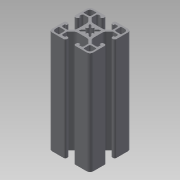
# Autodesk Inventor part: 40-4040-UL
Saved by Autodesk Inventor 2013 (Build 170138000, 138)
## iProperties
Created: 2014-04-23
Part Number: 40-4040-UL
Material: Generic
Document SubType Name: Modeling
Designer: Ross Bowman
Density: 1 g/cm^3
Engineer: Ross Bowman
Catalog Web Link: 8020.net
Vendor: 80/20 Inc.
Company: 80/20 Inc.
Author: Ross Bowman
Keywords: 80/20 , 8020 , T-Slot , Extrusion
Material: 6105-T5 Aluminum
Autodesk Inventor part; units mm, degrees
ref_plane "YZ Plane" through (0, 0, 0) normal (1, 0, 0) x (0, 1, 0)
ref_plane "XZ Plane" through (0, 0, 0) normal (0, 1, 0) x (-1, 0, 0)
ref_plane "XY Plane" through (0, 0, 0) normal (0, 0, 1) x (1, 0, 0)
sketch "Sketch1" plane through (0, 0, 0) normal (0, 0, 1) x (1, 0, 0)
  arc A0 (-5.4393, -4.8481) -> (-4.8481, -5.4393) centre (-4.9497, -4.9497) ccw
  line L0 (-5.1263, -3.712) -> (-5.4393, -4.8481)
  line L1 (-3.0049, -1.5907) -> (-5.1263, -3.712)
  arc A1 (-3.3421, -0.625) -> (-3.0049, -1.5907) centre (0, 0) ccw
  line L2 (-4.0876, -0.4923) -> (-3.3421, -0.625)
  arc A2 (-4.0876, 0.4923) -> (-4.0876, -0.4923) centre (-4, 0) ccw
  line L3 (-3.3421, 0.625) -> (-4.0876, 0.4923)
  arc A3 (-3.0049, 1.5907) -> (-3.3421, 0.625) centre (0, 0) ccw
  line L4 (-5.1263, 3.712) -> (-3.0049, 1.5907)
  line L5 (-5.4393, 4.8481) -> (-5.1263, 3.712)
  arc A4 (-4.8481, 5.4393) -> (-5.4393, 4.8481) centre (-4.9497, 4.9497) ccw
  line L6 (-3.712, 5.1263) -> (-4.8481, 5.4393)
  line L7 (-1.5907, 3.0049) -> (-3.712, 5.1263)
  arc A5 (-0.625, 3.3421) -> (-1.5907, 3.0049) centre (0, 0) ccw
  line L8 (-0.4923, 4.0876) -> (-0.625, 3.3421)
  arc A6 (0.4923, 4.0876) -> (-0.4923, 4.0876) centre (0, 4) ccw
  line L9 (0.625, 3.3421) -> (0.4923, 4.0876)
  arc A7 (1.5907, 3.0049) -> (0.625, 3.3421) centre (0, 0) ccw
  line L10 (3.712, 5.1263) -> (1.5907, 3.0049)
  line L11 (4.8481, 5.4393) -> (3.712, 5.1263)
  arc A8 (5.4393, 4.8481) -> (4.8481, 5.4393) centre (4.9497, 4.9497) ccw
  line L12 (5.1263, 3.712) -> (5.4393, 4.8481)
  line L13 (3.0049, 1.5907) -> (5.1263, 3.712)
  arc A9 (3.3421, 0.625) -> (3.0049, 1.5907) centre (0, 0) ccw
  line L14 (4.0876, 0.4923) -> (3.3421, 0.625)
  arc A10 (4.0876, -0.4923) -> (4.0876, 0.4923) centre (4, 0) ccw
  line L15 (3.3421, -0.625) -> (4.0876, -0.4923)
  arc A11 (3.0049, -1.5907) -> (3.3421, -0.625) centre (0, 0) ccw
  line L16 (5.1263, -3.712) -> (3.0049, -1.5907)
  line L17 (5.4393, -4.8481) -> (5.1263, -3.712)
  arc A12 (4.8481, -5.4393) -> (5.4393, -4.8481) centre (4.9497, -4.9497) ccw
  line L18 (3.712, -5.1263) -> (4.8481, -5.4393)
  line L19 (1.5907, -3.0049) -> (3.712, -5.1263)
  arc A13 (0.625, -3.3421) -> (1.5907, -3.0049) centre (0, 0) ccw
  line L20 (0.4923, -4.0876) -> (0.625, -3.3421)
  arc A14 (-0.4923, -4.0876) -> (0.4923, -4.0876) centre (0, -4) ccw
  line L21 (-0.625, -3.3421) -> (-0.4923, -4.0876)
  arc A15 (-1.5907, -3.0049) -> (-0.625, -3.3421) centre (0, 0) ccw
  line L22 (-3.712, -5.1263) -> (-1.5907, -3.0049)
  line L23 (-4.8481, -5.4393) -> (-3.712, -5.1263)
  arc A16 (-15.545, 18.345) -> (-18.345, 15.545) centre (-15.545, 15.545) ccw
  line L24 (-12.4898, 18.345) -> (-15.545, 18.345)
  arc A17 (-11.8598, 17.715) -> (-12.4898, 18.345) centre (-12.4898, 17.715) ccw
  line L25 (-11.8598, 13.1298) -> (-11.8598, 17.715)
  arc A18 (-13.1298, 11.8598) -> (-11.8598, 13.1298) centre (-13.1298, 13.1298) ccw
  line L26 (-17.715, 11.8598) -> (-13.1298, 11.8598)
  arc A19 (-18.345, 12.4898) -> (-17.715, 11.8598) centre (-17.715, 12.4898) ccw
  line L27 (-18.345, 15.545) -> (-18.345, 12.4898)
  arc A20 (18.345, 15.545) -> (15.545, 18.345) centre (15.545, 15.545) ccw
  line L28 (18.345, 12.4898) -> (18.345, 15.545)
  arc A21 (17.715, 11.8598) -> (18.345, 12.4898) centre (17.715, 12.4898) ccw
  line L29 (13.1298, 11.8598) -> (17.715, 11.8598)
  arc A22 (11.8598, 13.1298) -> (13.1298, 11.8598) centre (13.1298, 13.1298) ccw
  line L30 (11.8598, 17.715) -> (11.8598, 13.1298)
  arc A23 (12.4898, 18.345) -> (11.8598, 17.715) centre (12.4898, 17.715) ccw
  line L31 (15.545, 18.345) -> (12.4898, 18.345)
  arc A24 (-18.345, -15.545) -> (-15.545, -18.345) centre (-15.545, -15.545) ccw
  line L32 (-18.345, -12.4898) -> (-18.345, -15.545)
  arc A25 (-17.715, -11.8598) -> (-18.345, -12.4898) centre (-17.715, -12.4898) ccw
  line L33 (-13.1298, -11.8598) -> (-17.715, -11.8598)
  arc A26 (-11.8598, -13.1298) -> (-13.1298, -11.8598) centre (-13.1298, -13.1298) ccw
  line L34 (-11.8598, -17.715) -> (-11.8598, -13.1298)
  arc A27 (-12.4898, -18.345) -> (-11.8598, -17.715) centre (-12.4898, -17.715) ccw
  line L35 (-15.545, -18.345) -> (-12.4898, -18.345)
  arc A28 (15.545, -18.345) -> (18.345, -15.545) centre (15.545, -15.545) ccw
  line L36 (12.4898, -18.345) -> (15.545, -18.345)
  arc A29 (11.8598, -17.715) -> (12.4898, -18.345) centre (12.4898, -17.715) ccw
  line L37 (11.8598, -13.1298) -> (11.8598, -17.715)
  arc A30 (13.1298, -11.8598) -> (11.8598, -13.1298) centre (13.1298, -13.1298) ccw
  line L38 (17.715, -11.8598) -> (13.1298, -11.8598)
  arc A31 (18.345, -12.4898) -> (17.715, -11.8598) centre (17.715, -12.4898) ccw
  line L39 (18.345, -15.545) -> (18.345, -12.4898)
  arc A32 (-4.06, 18.43) -> (-5.63, 20) centre (-5.63, 18.43) ccw
  line L40 (-5.63, 20) -> (-16.83, 20)
  arc A33 (-16.83, 20) -> (-20, 16.83) centre (-16.83, 16.83) ccw
  line L41 (-20, 16.83) -> (-20, 5.63)
  arc A34 (-20, 5.63) -> (-18.43, 4.06) centre (-18.43, 5.63) ccw
  line L42 (-18.43, 4.06) -> (-17.57, 4.06)
  arc A35 (-17.57, 4.06) -> (-16, 5.63) centre (-17.57, 5.63) ccw
  line L43 (-16, 5.63) -> (-16, 6.605)
  arc A36 (-16, 6.605) -> (-16.25, 6.855) centre (-16.25, 6.605) ccw
  line L44 (-16.25, 6.855) -> (-17.25, 6.855)
  arc A37 (-17.5, 7.105) -> (-17.25, 6.855) centre (-17.25, 7.105) ccw
  line L45 (-17.5, 7.105) -> (-17.5, 9.015)
  arc A38 (-16.23, 10.285) -> (-17.5, 9.015) centre (-16.23, 9.015) ccw
  line L46 (-16.23, 10.285) -> (-12.2162, 10.285)
  arc A39 (-11.5869, 10.0243) -> (-12.2162, 10.285) centre (-12.2162, 9.395) ccw
  line L47 (-11.5869, 10.0243) -> (-9.0762, 7.5137)
  arc A40 (-7.685, 4.1549) -> (-9.0762, 7.5137) centre (-12.435, 4.1549) ccw
  line L48 (-7.685, 4.1549) -> (-7.685, -4.1549)
  arc A41 (-9.0762, -7.5137) -> (-7.685, -4.1549) centre (-12.435, -4.1549) ccw
  line L49 (-9.0762, -7.5137) -> (-11.5869, -10.0243)
  arc A42 (-12.2162, -10.285) -> (-11.5869, -10.0243) centre (-12.2162, -9.395) ccw
  line L50 (-12.2162, -10.285) -> (-16.23, -10.285)
  arc A43 (-17.5, -9.015) -> (-16.23, -10.285) centre (-16.23, -9.015) ccw
  line L51 (-17.5, -9.015) -> (-17.5, -7.105)
  arc A44 (-17.25, -6.855) -> (-17.5, -7.105) centre (-17.25, -7.105) ccw
  line L52 (-17.25, -6.855) -> (-16.25, -6.855)
  arc A45 (-16.25, -6.855) -> (-16, -6.605) centre (-16.25, -6.605) ccw
  line L53 (-16, -6.605) -> (-16, -5.63)
  arc A46 (-16, -5.63) -> (-17.57, -4.06) centre (-17.57, -5.63) ccw
  line L54 (-17.57, -4.06) -> (-18.43, -4.06)
  arc A47 (-18.43, -4.06) -> (-20, -5.63) centre (-18.43, -5.63) ccw
  line L55 (-20, -5.63) -> (-20, -16.83)
  arc A48 (-20, -16.83) -> (-16.83, -20) centre (-16.83, -16.83) ccw
  line L56 (-16.83, -20) -> (-5.63, -20)
  arc A49 (-5.63, -20) -> (-4.06, -18.43) centre (-5.63, -18.43) ccw
  line L57 (-4.06, -18.43) -> (-4.06, -17.57)
  arc A50 (-4.06, -17.57) -> (-5.63, -16) centre (-5.63, -17.57) ccw
  line L58 (-5.63, -16) -> (-6.605, -16)
  arc A51 (-6.605, -16) -> (-6.855, -16.25) centre (-6.605, -16.25) ccw
  line L59 (-6.855, -16.25) -> (-6.855, -17.25)
  arc A52 (-7.105, -17.5) -> (-6.855, -17.25) centre (-7.105, -17.25) ccw
  line L60 (-7.105, -17.5) -> (-9.015, -17.5)
  arc A53 (-10.285, -16.23) -> (-9.015, -17.5) centre (-9.015, -16.23) ccw
  line L61 (-10.285, -16.23) -> (-10.285, -12.2162)
  arc A54 (-10.0243, -11.5869) -> (-10.285, -12.2162) centre (-9.395, -12.2162) ccw
  line L62 (-10.0243, -11.5869) -> (-7.5137, -9.0762)
  arc A55 (-4.1549, -7.685) -> (-7.5137, -9.0762) centre (-4.1549, -12.435) ccw
  line L63 (-4.1549, -7.685) -> (4.1549, -7.685)
  arc A56 (7.5137, -9.0762) -> (4.1549, -7.685) centre (4.1549, -12.435) ccw
  line L64 (7.5137, -9.0762) -> (10.0243, -11.5869)
  arc A57 (10.285, -12.2162) -> (10.0243, -11.5869) centre (9.395, -12.2162) ccw
  line L65 (10.285, -12.2162) -> (10.285, -16.23)
  arc A58 (9.015, -17.5) -> (10.285, -16.23) centre (9.015, -16.23) ccw
  line L66 (9.015, -17.5) -> (7.105, -17.5)
  arc A59 (6.855, -17.25) -> (7.105, -17.5) centre (7.105, -17.25) ccw
  line L67 (6.855, -17.25) -> (6.855, -16.25)
  arc A60 (6.855, -16.25) -> (6.605, -16) centre (6.605, -16.25) ccw
  line L68 (6.605, -16) -> (5.63, -16)
  arc A61 (5.63, -16) -> (4.06, -17.57) centre (5.63, -17.57) ccw
  line L69 (4.06, -17.57) -> (4.06, -18.43)
  arc A62 (4.06, -18.43) -> (5.63, -20) centre (5.63, -18.43) ccw
  line L70 (5.63, -20) -> (16.83, -20)
  arc A63 (16.83, -20) -> (20, -16.83) centre (16.83, -16.83) ccw
  line L71 (20, -16.83) -> (20, -5.63)
  arc A64 (20, -5.63) -> (18.43, -4.06) centre (18.43, -5.63) ccw
  line L72 (18.43, -4.06) -> (17.57, -4.06)
  arc A65 (17.57, -4.06) -> (16, -5.63) centre (17.57, -5.63) ccw
  line L73 (16, -5.63) -> (16, -6.605)
  arc A66 (16, -6.605) -> (16.25, -6.855) centre (16.25, -6.605) ccw
  line L74 (16.25, -6.855) -> (17.25, -6.855)
  arc A67 (17.5, -7.105) -> (17.25, -6.855) centre (17.25, -7.105) ccw
  line L75 (17.5, -7.105) -> (17.5, -9.015)
  arc A68 (16.23, -10.285) -> (17.5, -9.015) centre (16.23, -9.015) ccw
  line L76 (16.23, -10.285) -> (12.2162, -10.285)
  arc A69 (11.5869, -10.0243) -> (12.2162, -10.285) centre (12.2162, -9.395) ccw
  line L77 (11.5869, -10.0243) -> (9.0762, -7.5137)
  arc A70 (7.685, -4.1549) -> (9.0762, -7.5137) centre (12.435, -4.1549) ccw
  line L78 (7.685, -4.1549) -> (7.685, 4.1549)
  arc A71 (9.0762, 7.5137) -> (7.685, 4.1549) centre (12.435, 4.1549) ccw
  line L79 (9.0762, 7.5137) -> (11.5869, 10.0243)
  arc A72 (12.2162, 10.285) -> (11.5869, 10.0243) centre (12.2162, 9.395) ccw
  line L80 (12.2162, 10.285) -> (16.23, 10.285)
  arc A73 (17.5, 9.015) -> (16.23, 10.285) centre (16.23, 9.015) ccw
  line L81 (17.5, 9.015) -> (17.5, 7.105)
  arc A74 (17.25, 6.855) -> (17.5, 7.105) centre (17.25, 7.105) ccw
  line L82 (17.25, 6.855) -> (16.25, 6.855)
  arc A75 (16.25, 6.855) -> (16, 6.605) centre (16.25, 6.605) ccw
  line L83 (16, 6.605) -> (16, 5.63)
  arc A76 (16, 5.63) -> (17.57, 4.06) centre (17.57, 5.63) ccw
  line L84 (17.57, 4.06) -> (18.43, 4.06)
  arc A77 (18.43, 4.06) -> (20, 5.63) centre (18.43, 5.63) ccw
  line L85 (20, 5.63) -> (20, 16.83)
  arc A78 (20, 16.83) -> (16.83, 20) centre (16.83, 16.83) ccw
  line L86 (16.83, 20) -> (5.63, 20)
  arc A79 (5.63, 20) -> (4.06, 18.43) centre (5.63, 18.43) ccw
  line L87 (4.06, 18.43) -> (4.06, 17.57)
  arc A80 (4.06, 17.57) -> (5.63, 16) centre (5.63, 17.57) ccw
  line L88 (5.63, 16) -> (6.605, 16)
  arc A81 (6.605, 16) -> (6.855, 16.25) centre (6.605, 16.25) ccw
  line L89 (6.855, 16.25) -> (6.855, 17.25)
  arc A82 (7.105, 17.5) -> (6.855, 17.25) centre (7.105, 17.25) ccw
  line L90 (7.105, 17.5) -> (9.015, 17.5)
  arc A83 (10.285, 16.23) -> (9.015, 17.5) centre (9.015, 16.23) ccw
  line L91 (10.285, 16.23) -> (10.285, 12.2162)
  arc A84 (10.0243, 11.5869) -> (10.285, 12.2162) centre (9.395, 12.2162) ccw
  line L92 (10.0243, 11.5869) -> (7.5137, 9.0762)
  arc A85 (4.1549, 7.685) -> (7.5137, 9.0762) centre (4.1549, 12.435) ccw
  line L93 (4.1549, 7.685) -> (-4.1549, 7.685)
  arc A86 (-7.5137, 9.0762) -> (-4.1549, 7.685) centre (-4.1549, 12.435) ccw
  line L94 (-7.5137, 9.0762) -> (-10.0243, 11.5869)
  arc A87 (-10.285, 12.2162) -> (-10.0243, 11.5869) centre (-9.395, 12.2162) ccw
  line L95 (-10.285, 12.2162) -> (-10.285, 16.23)
  arc A88 (-9.015, 17.5) -> (-10.285, 16.23) centre (-9.015, 16.23) ccw
  line L96 (-9.015, 17.5) -> (-7.105, 17.5)
  arc A89 (-6.855, 17.25) -> (-7.105, 17.5) centre (-7.105, 17.25) ccw
  line L97 (-6.855, 17.25) -> (-6.855, 16.25)
  arc A90 (-6.855, 16.25) -> (-6.605, 16) centre (-6.605, 16.25) ccw
  line L98 (-6.605, 16) -> (-5.63, 16)
  arc A91 (-5.63, 16) -> (-4.06, 17.57) centre (-5.63, 17.57) ccw
  line L99 (-4.06, 17.57) -> (-4.06, 18.43)
  constraints: 200 end point, 184 point on circle, 92 centre point
extrude "Extrusion1" add sketch "Sketch1" against normal blind 100
body "Solid1"
